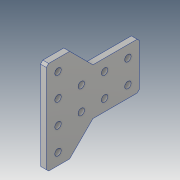
# Autodesk Inventor part: 200-40-BOGIE-CONNECTOR-06
Saved by Autodesk Inventor 2018.2 (Build 222227000, 227)
## iProperties
Manager: feesmrt
Company: FRANCOR
Part Number: 200-40-BOGIE-CONNECTOR-06
Project: Rescue Robot
Cost Center: -
Material: Aluminium 6061
Document SubType Name: Modeling
Designer: feesmrt
Engineer: feesmrt
Authority: feesmrt
Density: 2.7 g/cm^3
Appearance: Aluminium - flach
Description: Bogie Connector Verstärkungsplatte
Stock Number: 200-40-BOGIE-CONNECTOR-06
Mass: 165.052 g
Surface Area: 105.648 cm^2
Volume: 20.6315 cm^3
Subject: Rescue Robot
Author: feesmrt
Revision Number: 1
Title: Bogie Connector Verstärkungsplatte
Autodesk Inventor part; units mm, degrees
ref_plane "YZ Plane" through (0, 0, 0) normal (1, 0, 0) x (0, 1, 0)
ref_plane "XZ Plane" through (0, 0, 0) normal (0, 1, 0) x (-1, 0, 0)
ref_plane "XY Plane" through (0, 0, 0) normal (0, 0, 1) x (1, 0, 0)
sketch "Skizze1" plane through (0, 0, 0) normal (1, 0, 0) x (0, 1, 0)
  line L0 (0, 56) -> (0, -56) construction
  line L1 (-56, 0) -> (56, 0) construction
  line L2 (-40, 40) -> (-40, -40)
  line L3 (40, 20) -> (40, -20)
  line L4 (-40, 40) -> (-20, 40)
  line L5 (-20, 40) -> (0, 20)
  line L6 (0, 20) -> (40, 20)
  line L7 (-40, -40) -> (-20, -40)
  line L8 (-20, -40) -> (0, -20)
  line L9 (0, -20) -> (40, -20)
  point P0 (0, 0)
  dimension "d21" = 80
  dimension "d22" = 40
  dimension "d23" = 20
  dimension "d24" = 20
  dimension "d25" = 80
  constraints: 16 end point, 4 symmetric about line, 2 perpendicular, 1 horizontal, 1 vertical, 1 other
  measures "d21" distance of L2.start L2.end
  measures "d22" distance of L3.start L3.end
  measures "d23" distance of L2.start L4.end
  measures "d24" horizontal distance of L4.end L5.end
  measures "d25" distance between parallel lines of L2 L3
extrude "Grundkörper" add sketch "Skizze1" along normal mid plane 5
sketch "Skizze3" plane through (2.5, 0, 0) normal (1, 0, 0) x (0, 0, -1)
  line L0 (-40, -40) -> (40, -40) construction
  line L1 (-40, -20) -> (-40, -40) construction
  line L2 (40, -40) -> (40, -20) construction
  line L3 (40, -20) -> (20, 0) construction
  line L4 (20, 0) -> (20, 40) construction
  line L5 (20, 40) -> (-20, 40) construction
  line L6 (-20, 40) -> (-20, 0) construction
  line L7 (-20, 0) -> (-40, -20) construction
  line L8 (-40, -40) -> (-40, -20) projected
  line L9 (-40, -30) -> (40, -30) construction
  line L10 (-56, 0) -> (56, 0) construction
  line L11 (0, -56) -> (0, 56) construction
  line L12 (-10, 40) -> (-10, 0) construction
  line L13 (-20, 20) -> (20, 20) construction
  point P0 (0, 0)
  point P1 (-10, -30)
  point P2 (-30, -30)
  point P3 (10, -30)
  point P4 (30, -30)
  point P5 (-10, 10)
  point P6 (-10, 30)
  point P7 (10, 10)
  point P8 (10, 30)
  point P9 (-10, -10)
  point P10 (10, -10)
  dimension "d27" = 20
  dimension "d28" = 20
  dimension "d29" = 10
  dimension "d30" = 40
  dimension "d31" = 20
  dimension "d42" = 20
  constraints: 7 point on line, 6 end point, 6 symmetric about line, 4 midpoint, 2 perpendicular
  measures "d27" distance of point (-30, -30) point (-10, -30)
  measures "d28" distance of point (-10, -30) point (10, -30)
  measures "d29" distance between parallel lines of L11 L12
  measures "d30" distance between parallel lines of L6 L4
  measures "d31" distance of point (-10, 30) point (-10, 10)
  measures "d42" distance of point (-10, 10) point (-10, -10)
hole "BOH_M5" at (2.5, -30, 10) at (2.5, -30, 30) at (2.5, -30, -30) at (2.5, -30, -10) at (2.5, 10, 10) at (2.5, 30, 10) at (2.5, 10, -10) at (2.5, 30, -10) at (2.5, -10, 10) at (2.5, -10, -10) direction (-1, 0, 0) diameter 5.5 end through all
chamfer "FASE_Allgemein" distance 2 angle 45 4 edges at (0, -40, 40) (0, 40, 20) (0, -40, -40) (0, 40, -20)
equation "\"d27\" = d28"
equation "\"d28\" = 0.5 * d30"
equation "\"d29\" = 0.25 * d30"
equation "\"d31\" = d27"
equation "\"d42\" = d31"
